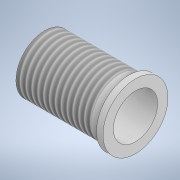
# Autodesk Inventor part: 2.2
Saved by Autodesk Inventor 2020 (Build 240168000, 168)
## iProperties
Created: 2022-04-20
Part Number: 2.2
Material: Типовые
Document SubType Name: Modeling
Designer: User
Density: 1 g/cm^3
Appearance: По умолчанию
Author: User
Autodesk Inventor part; units mm, degrees
ref_plane "YZ Plane" through (0, 0, 0) normal (1, 0, 0) x (0, 1, 0)
ref_plane "XZ Plane" through (0, 0, 0) normal (0, 1, 0) x (-1, 0, 0)
ref_plane "XY Plane" through (0, 0, 0) normal (0, 0, 1) x (1, 0, 0)
sketch "Эскиз1" plane through (0, 0, 0) normal (0, 0, 1) x (1, 0, 0)
  line L0 (0, 0) -> (100, 0)
  line L1 (0, 0) -> (0, 30)
  line L2 (0, 30) -> (60, 30)
  line L3 (60, 30) -> (60, 0)
  line L4 (100, 0) -> (100, 25)
  line L5 (100, 25) -> (95, 25)
  line L6 (95, 25) -> (95, 22)
  line L7 (95, 22) -> (25, 22)
  line L8 (25, 22) -> (25, 25)
  line L9 (25, 25) -> (20, 25)
  line L10 (20, 25) -> (20, 0)
  line L11 (0, 20) -> (10, 20)
  line L12 (10, 20) -> (10, 17)
  line L13 (10, 17) -> (20, 17)
  line L14 (30, 22) -> (30, 17)
  line L15 (30, 17) -> (100, 17)
  line L16 (10, 17) -> (0, 17)
  line L17 (87.9599, 22) -> (87.9599, 19.5)
  line L18 (87.9599, 19.5) -> (25, 19.5)
  line L19 (25, 19.5) -> (25, 22)
  point P0 (60, 22)
  point P1 (60, 19.5)
  dimension "d0" = 100
  dimension "d1" = 30
  dimension "d2" = 60
  dimension "d3" = 25
  dimension "d4" = 5
  dimension "d5" = 3
  dimension "d6" = 70
  dimension "d7" = 3
  dimension "d8" = 5
  dimension "d9" = 10
  dimension "d10" = 3
  dimension "d11" = 8
  dimension "d12" = 70
  dimension "d13" = 8
  dimension "d14" = 40
  dimension "d15" = 5
  dimension "d16" = 12.0401
  dimension "d17" = 5.5
  constraints: 40 end point, 12 perpendicular, 10 point on line, 4 vertical, 1 horizontal, 1 parallel
  measures "d0" distance of L0.start L0.end
  measures "d1" distance of L0.start L1.end
  measures "d2" distance of L1.end L2.end
  measures "d3" distance of L0.end L4.end
  measures "d4" distance of L4.end L5.end
  measures "d5" distance of L5.end L6.end
  measures "d6" distance of L6.end L7.end
  measures "d7" distance of L7.end L8.end
  measures "d8" distance of L8.end L9.end
  measures "d9" distance of L11.start L11.end
  measures "d10" distance of L11.end L12.end
  measures "d11" distance between parallel lines of L9 L13
  measures "d12" distance between parallel lines of L14 L4
  measures "d13" distance between parallel lines of L15 L5
  measures "d14" distance from line of point (60, 22) L4
  measures "d15" distance from line of point (60, 22) L15
  measures "d16" distance between parallel lines of L17 L4
  measures "d17" distance between parallel lines of L18 L5
revolve "Вращение1" add sketch "Эскиз1" angle 360 about axis through (0, 0, 0) along (1, 0, 0) contours L15 L14 L18 L3 | L3 L18 L17 L7 L6 L5 L4 L15 | L18 L14 L7 L3 | L3 L7 L17 L18
thread "Резьба1" size "M45x4.5" class "6g" standard "ANSI Metric M Profile" length 58
